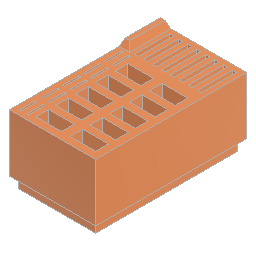
Online-Storage-Carrier (Autodesk Fusion 360 design; units mm, degrees)
Autodesk Fusion 360 part; units mm, degrees
sketch "Sketch1" plane through (0, 0, 18.175) normal (0, 0, 1) x (-1, 0, 0)
  line L0 (-2.95, 294.992) -> (-2.95, 195.892)
  line L1 (-2.95, 195.892) -> (-57.05, 195.892)
  line L2 (-57.05, 195.892) -> (-57.05, 294.992)
  line L3 (-57.05, 294.992) -> (-2.95, 294.992)
  line L4 (0, 192.942) -> (0, 297.942)
  line L5 (0, 297.942) -> (-60, 297.942)
  line L6 (-60, 297.942) -> (-60, 192.942)
  line L7 (-60, 192.942) -> (0, 192.942)
  line L8 (0, 297.942) -> (-60, 297.942)
  line L9 (-60, 297.942) -> (-60, 192.942)
  line L10 (-60, 192.942) -> (0, 192.942)
  line L11 (0, 192.942) -> (0, 297.942)
  line L12 (-56.95, 294.892) -> (-56.95, 195.992)
  line L13 (-56.95, 195.992) -> (-3.05, 195.992)
  line L14 (-3.05, 195.992) -> (-3.05, 294.892)
  line L15 (-3.05, 294.892) -> (-56.95, 294.892)
  point P0 (0, 297.942)
  dimension "d14" = 60
  dimension "d15" = 105
  dimension "d17" = 0.1
  constraint horizontal L8
  constraint vertical L9
  constraint horizontal L10
  constraint vertical L11
  constraint coincident P0 L4.end
  measures "d14" distance of P0 L5.end
  measures "d15" distance of P0 L4.start
  measures "d17" distance of L0 L14
extrude "Extrude1" add sketch "Sketch1" against normal blind 7.5 contours L12 L13 L14 L15
sketch "Sketch2" plane through (0, 0, 18.175) normal (0, 0, 1) x (-1, 0, 0)
  line L0 (-3.05, 294.892) -> (-56.95, 294.892)
  line L1 (-56.95, 294.892) -> (-56.95, 195.992)
  line L2 (-56.95, 195.992) -> (-3.05, 195.992)
  line L3 (-3.05, 195.992) -> (-3.05, 294.892)
  line L4 (0, 297.942) -> (-60, 297.942)
  line L5 (-60, 297.942) -> (-60, 192.942)
  line L6 (-60, 192.942) -> (0, 192.942)
  line L7 (0, 192.942) -> (0, 297.942)
  point P0 (0, 297.942)
  dimension "d21" = 60
  dimension "d22" = 105
  constraint horizontal L4
  constraint vertical L5
  constraint horizontal L6
  constraint vertical L7
  constraint coincident P0 L4.start
  measures "d21" distance of P0 L4.end
  measures "d22" distance of P0 L6.end
extrude "Extrude2" add sketch "Sketch2" along normal blind 40 contours L0 L1 L2 L3 | L4 L5 L6 L7
sketch "Sketch3" plane through (0, 0, 58.175) normal (0, 0, 1) x (-1, 0, 0)
  line L0 (0, 192.942) -> (0, 297.942)
  line L1 (0, 297.942) -> (-60, 297.942)
  line L2 (-60, 297.942) -> (-60, 192.942)
  line L3 (-60, 192.942) -> (0, 192.942)
  line L4 (-55, 284.142) -> (-37.2, 284.142)
  line L5 (-37.2, 284.142) -> (-37.2, 292.942)
  line L6 (-37.2, 292.942) -> (-55, 292.942)
  line L7 (-55, 292.942) -> (-55, 284.142)
  line L8 (-60, 224.192) -> (0, 224.192)
  line L9 (-55, 270.342) -> (-37.2, 270.342)
  line L10 (-37.2, 270.342) -> (-37.2, 279.142)
  line L11 (-37.2, 279.142) -> (-55, 279.142)
  line L12 (-55, 279.142) -> (-55, 270.342)
  line L13 (-55, 256.542) -> (-37.2, 256.542)
  line L14 (-37.2, 256.542) -> (-37.2, 265.342)
  line L15 (-37.2, 265.342) -> (-55, 265.342)
  line L16 (-55, 265.342) -> (-55, 256.542)
  line L17 (-55, 242.742) -> (-37.2, 242.742)
  line L18 (-37.2, 242.742) -> (-37.2, 251.542)
  line L19 (-37.2, 251.542) -> (-55, 251.542)
  line L20 (-55, 251.542) -> (-55, 242.742)
  line L21 (-55, 228.942) -> (-37.2, 228.942)
  line L22 (-37.2, 228.942) -> (-37.2, 237.742)
  line L23 (-37.2, 237.742) -> (-55, 237.742)
  line L24 (-55, 237.742) -> (-55, 228.942)
  line L25 (-31.2, 284.142) -> (-13.4, 284.142)
  line L26 (-13.4, 284.142) -> (-13.4, 292.942)
  line L27 (-13.4, 292.942) -> (-31.2, 292.942)
  line L28 (-31.2, 292.942) -> (-31.2, 284.142)
  line L29 (-31.2, 270.342) -> (-13.4, 270.342)
  line L30 (-13.4, 270.342) -> (-13.4, 279.142)
  line L31 (-13.4, 279.142) -> (-31.2, 279.142)
  line L32 (-31.2, 279.142) -> (-31.2, 270.342)
  line L33 (-31.2, 256.542) -> (-13.4, 256.542)
  line L34 (-13.4, 256.542) -> (-13.4, 265.342)
  line L35 (-13.4, 265.342) -> (-31.2, 265.342)
  line L36 (-31.2, 265.342) -> (-31.2, 256.542)
  line L37 (-31.2, 242.742) -> (-13.4, 242.742)
  line L38 (-13.4, 242.742) -> (-13.4, 251.542)
  line L39 (-13.4, 251.542) -> (-31.2, 251.542)
  line L40 (-31.2, 251.542) -> (-31.2, 242.742)
  line L41 (-31.2, 228.942) -> (-13.4, 228.942)
  line L42 (-13.4, 228.942) -> (-13.4, 237.742)
  line L43 (-13.4, 237.742) -> (-31.2, 237.742)
  line L44 (-31.2, 237.742) -> (-31.2, 228.942)
  dimension "d33" = 17.8
  dimension "d34" = 8.8
  dimension "d35" = 5
  dimension "d36" = 5
  dimension "d38" = 73.75
  dimension "d39" = 31.25
  dimension "d42" = 13.8
  dimension "d43" = 23.8
  dimension "d44" = 4.75
  dimension "d45" = 5
  dimension "d46" = 6
  constraint horizontal L4
  constraint vertical L5
  constraint horizontal L6
  constraint vertical L7
  constraint coincident L2 L8.start
  constraint coincident L0 L8.end
  constraint perpendicular L0 L8
  measures "d33" distance of L4.start L4.end
  measures "d34" distance of L4.start L6.end
  measures "d35" distance of L1 L6
  measures "d36" distance of L2 L7
  measures "d38" distance of L1 L8
  measures "d39" distance of L3 L8
  measures "d44" distance of L8 L21
  measures "d45" distance of L17 L23
  measures "d46" distance of L22 L44
extrude "Extrude3" cut sketch "Sketch3" against normal blind 37.5 contours L4 L5 L6 L7 | L9 L10 L11 L12 | L13 L14 L15 L16 | L17 L18 L19 L20 | L21 L22 L23 L24 | L25 L26 L27 L28 | L29 L30 L31 L32 | L33 L34 L35 L36 | L37 L38 L39 L40 | L41 L42 L43 L44
sketch "Sketch4" plane through (0, 0, 58.175) normal (0, 0, 1) x (-1, 0, 0)
  line L0 (-37.2, 242.742) -> (-55, 242.742)
  line L1 (-55, 242.742) -> (-55, 251.542)
  line L2 (-55, 251.542) -> (-37.2, 251.542)
  line L3 (-37.2, 251.542) -> (-37.2, 242.742)
  line L4 (-37.2, 270.342) -> (-55, 270.342)
  line L5 (-55, 270.342) -> (-55, 279.142)
  line L6 (-55, 279.142) -> (-37.2, 279.142)
  line L7 (-37.2, 279.142) -> (-37.2, 270.342)
  line L8 (-37.2, 284.142) -> (-55, 284.142)
  line L9 (-55, 284.142) -> (-55, 292.942)
  line L10 (-55, 292.942) -> (-37.2, 292.942)
  line L11 (-37.2, 292.942) -> (-37.2, 284.142)
  line L12 (-37.2, 256.542) -> (-55, 256.542)
  line L13 (-55, 256.542) -> (-55, 265.342)
  line L14 (-55, 265.342) -> (-37.2, 265.342)
  line L15 (-37.2, 265.342) -> (-37.2, 256.542)
  line L16 (-37.2, 228.942) -> (-55, 228.942)
  line L17 (-55, 228.942) -> (-55, 237.742)
  line L18 (-55, 237.742) -> (-37.2, 237.742)
  line L19 (-37.2, 237.742) -> (-37.2, 228.942)
  line L20 (-13.4, 242.742) -> (-31.2, 242.742)
  line L21 (-31.2, 242.742) -> (-31.2, 251.542)
  line L22 (-31.2, 251.542) -> (-13.4, 251.542)
  line L23 (-13.4, 251.542) -> (-13.4, 242.742)
  line L24 (-13.4, 270.342) -> (-31.2, 270.342)
  line L25 (-31.2, 270.342) -> (-31.2, 279.142)
  line L26 (-31.2, 279.142) -> (-13.4, 279.142)
  line L27 (-13.4, 279.142) -> (-13.4, 270.342)
  line L28 (-13.4, 284.142) -> (-31.2, 284.142)
  line L29 (-31.2, 284.142) -> (-31.2, 292.942)
  line L30 (-31.2, 292.942) -> (-13.4, 292.942)
  line L31 (-13.4, 292.942) -> (-13.4, 284.142)
  line L32 (-13.4, 256.542) -> (-31.2, 256.542)
  line L33 (-31.2, 256.542) -> (-31.2, 265.342)
  line L34 (-31.2, 265.342) -> (-13.4, 265.342)
  line L35 (-13.4, 265.342) -> (-13.4, 256.542)
  line L36 (-13.4, 228.942) -> (-31.2, 228.942)
  line L37 (-31.2, 228.942) -> (-31.2, 237.742)
  line L38 (-31.2, 237.742) -> (-13.4, 237.742)
  line L39 (-13.4, 237.742) -> (-13.4, 228.942)
  line L40 (0, 192.942) -> (0, 297.942)
  line L41 (0, 297.942) -> (-60, 297.942)
  line L42 (-60, 297.942) -> (-60, 192.942)
  line L43 (-60, 192.942) -> (0, 192.942)
  line L44 (-53.75, 196.442) -> (-56.5, 196.442)
  line L45 (-56.5, 196.442) -> (-56.5, 220.942)
  line L46 (-56.5, 220.942) -> (-53.75, 220.942)
  line L47 (-53.75, 220.942) -> (-53.75, 196.442)
  line L48 (-47.5, 196.442) -> (-50.25, 196.442)
  line L49 (-47.5, 220.942) -> (-47.5, 196.442)
  line L50 (-50.25, 196.442) -> (-50.25, 220.942)
  line L51 (-50.25, 220.942) -> (-47.5, 220.942)
  line L52 (-41.25, 196.442) -> (-44, 196.442)
  line L53 (-41.25, 220.942) -> (-41.25, 196.442)
  line L54 (-44, 196.442) -> (-44, 220.942)
  line L55 (-44, 220.942) -> (-41.25, 220.942)
  line L56 (-35, 196.442) -> (-37.75, 196.442)
  line L57 (-35, 220.942) -> (-35, 196.442)
  line L58 (-37.75, 196.442) -> (-37.75, 220.942)
  line L59 (-37.75, 220.942) -> (-35, 220.942)
  line L60 (-28.75, 196.442) -> (-31.5, 196.442)
  line L61 (-28.75, 220.942) -> (-28.75, 196.442)
  line L62 (-31.5, 196.442) -> (-31.5, 220.942)
  line L63 (-31.5, 220.942) -> (-28.75, 220.942)
  line L64 (-22.5, 196.442) -> (-25.25, 196.442)
  line L65 (-22.5, 220.942) -> (-22.5, 196.442)
  line L66 (-25.25, 196.442) -> (-25.25, 220.942)
  line L67 (-25.25, 220.942) -> (-22.5, 220.942)
  line L68 (-16.25, 196.442) -> (-19, 196.442)
  line L69 (-16.25, 220.942) -> (-16.25, 196.442)
  line L70 (-19, 196.442) -> (-19, 220.942)
  line L71 (-19, 220.942) -> (-16.25, 220.942)
  line L72 (-10, 196.442) -> (-12.75, 196.442)
  line L73 (-10, 220.942) -> (-10, 196.442)
  line L74 (-12.75, 196.442) -> (-12.75, 220.942)
  line L75 (-12.75, 220.942) -> (-10, 220.942)
  dimension "d51" = 2.75
  dimension "d52" = 24.5
  dimension "d54" = 3.5
  dimension "d55" = 3.5
  dimension "d65" = 6.25
  dimension "d66" = 0
  constraint horizontal L44
  constraint vertical L45
  constraint horizontal L46
  constraint vertical L47
  measures "d51" distance of L44.start L44.end
  measures "d52" distance of L44.start L46.end
  measures "d54" distance of L43 L44
  measures "d55" distance of L42 L45
sketch "Sketch5" plane through (0, 0, 58.175) normal (0, 0, 1) x (-1, 0, 0)
  line L0 (-37.2, 242.742) -> (-55, 242.742)
  line L1 (-55, 242.742) -> (-55, 251.542)
  line L2 (-55, 251.542) -> (-37.2, 251.542)
  line L3 (-37.2, 251.542) -> (-37.2, 242.742)
  line L4 (-37.2, 270.342) -> (-55, 270.342)
  line L5 (-55, 270.342) -> (-55, 279.142)
  line L6 (-55, 279.142) -> (-37.2, 279.142)
  line L7 (-37.2, 279.142) -> (-37.2, 270.342)
  line L8 (-37.2, 284.142) -> (-55, 284.142)
  line L9 (-55, 284.142) -> (-55, 292.942)
  line L10 (-55, 292.942) -> (-37.2, 292.942)
  line L11 (-37.2, 292.942) -> (-37.2, 284.142)
  line L12 (-37.2, 256.542) -> (-55, 256.542)
  line L13 (-55, 256.542) -> (-55, 265.342)
  line L14 (-55, 265.342) -> (-37.2, 265.342)
  line L15 (-37.2, 265.342) -> (-37.2, 256.542)
  line L16 (-37.2, 228.942) -> (-55, 228.942)
  line L17 (-55, 228.942) -> (-55, 237.742)
  line L18 (-55, 237.742) -> (-37.2, 237.742)
  line L19 (-37.2, 237.742) -> (-37.2, 228.942)
  line L20 (-13.4, 242.742) -> (-31.2, 242.742)
  line L21 (-31.2, 242.742) -> (-31.2, 251.542)
  line L22 (-31.2, 251.542) -> (-13.4, 251.542)
  line L23 (-13.4, 251.542) -> (-13.4, 242.742)
  line L24 (-13.4, 270.342) -> (-31.2, 270.342)
  line L25 (-31.2, 270.342) -> (-31.2, 279.142)
  line L26 (-31.2, 279.142) -> (-13.4, 279.142)
  line L27 (-13.4, 279.142) -> (-13.4, 270.342)
  line L28 (-13.4, 284.142) -> (-31.2, 284.142)
  line L29 (-31.2, 284.142) -> (-31.2, 292.942)
  line L30 (-31.2, 292.942) -> (-13.4, 292.942)
  line L31 (-13.4, 292.942) -> (-13.4, 284.142)
  line L32 (-13.4, 256.542) -> (-31.2, 256.542)
  line L33 (-31.2, 256.542) -> (-31.2, 265.342)
  line L34 (-31.2, 265.342) -> (-13.4, 265.342)
  line L35 (-13.4, 265.342) -> (-13.4, 256.542)
  line L36 (-13.4, 228.942) -> (-31.2, 228.942)
  line L37 (-31.2, 228.942) -> (-31.2, 237.742)
  line L38 (-31.2, 237.742) -> (-13.4, 237.742)
  line L39 (-13.4, 237.742) -> (-13.4, 228.942)
  line L40 (0, 192.942) -> (0, 297.942)
  line L41 (0, 297.942) -> (-60, 297.942)
  line L42 (-60, 297.942) -> (-60, 192.942)
  line L43 (-60, 192.942) -> (0, 192.942)
  line L44 (0, 192.942) -> (-7.25, 192.942)
  line L45 (-7.25, 192.942) -> (-7.25, 221.442)
  line L46 (-7.25, 221.442) -> (0, 221.442)
  line L47 (0, 221.442) -> (0, 192.942)
  dimension "d56" = 7.25
  dimension "d57" = 28.5
  constraint horizontal L44
  constraint vertical L45
  constraint horizontal L46
  constraint vertical L47
  constraint coincident L40.start L43.end
  measures "d56" distance of L40.start L44.end
  measures "d57" distance of L40.start L46.end
extrude "Extrude4" add sketch "Sketch5" along normal blind 3 contours L40 L43 L44 L45 L46 L47
chamfer "Chamfer1" distance 4 distance2 3 2 edges at (7.25, -207.192, 61.175) (3.625, -221.442, 61.175) measured on face at (2.4167, -211.942, 61.175) measured on face at (2.4167, -211.942, 61.175)
extrude "Extrude5" cut sketch "Sketch4" against normal blind 21 contours L44 L45 L46 L47 | L48 L49 L50 L51 | L52 L53 L54 L55 | L56 L57 L58 L59 | L60 L61 L62 L63 | L64 L65 L66 L67 | L68 L69 L70 L71 | L72 L73 L74 L75
sketch "Sketch1 (2)" plane through (0, 0, 58.175) normal (0, 0, 1) x (-1, 0, 0)
  line L0 (-22.5, 196.442) -> (-25.25, 196.442)
  line L1 (-25.25, 196.442) -> (-25.25, 220.942)
  line L2 (-25.25, 220.942) -> (-22.5, 220.942)
  line L3 (-22.5, 220.942) -> (-22.5, 196.442)
  line L4 (-47.5, 196.442) -> (-50.25, 196.442)
  line L5 (-50.25, 196.442) -> (-50.25, 220.942)
  line L6 (-50.25, 220.942) -> (-47.5, 220.942)
  line L7 (-47.5, 220.942) -> (-47.5, 196.442)
  line L8 (-41.25, 196.442) -> (-44, 196.442)
  line L9 (-44, 196.442) -> (-44, 220.942)
  line L10 (-44, 220.942) -> (-41.25, 220.942)
  line L11 (-41.25, 220.942) -> (-41.25, 196.442)
  line L12 (-16.25, 196.442) -> (-19, 196.442)
  line L13 (-19, 196.442) -> (-19, 220.942)
  line L14 (-19, 220.942) -> (-16.25, 220.942)
  line L15 (-16.25, 220.942) -> (-16.25, 196.442)
  line L16 (-28.75, 196.442) -> (-31.5, 196.442)
  line L17 (-31.5, 196.442) -> (-31.5, 220.942)
  line L18 (-31.5, 220.942) -> (-28.75, 220.942)
  line L19 (-28.75, 220.942) -> (-28.75, 196.442)
  line L20 (-56.5, 196.442) -> (-56.5, 220.942)
  line L21 (-56.5, 220.942) -> (-53.75, 220.942)
  line L22 (-53.75, 220.942) -> (-53.75, 196.442)
  line L23 (-53.75, 196.442) -> (-56.5, 196.442)
  line L24 (-35, 196.442) -> (-37.75, 196.442)
  line L25 (-37.75, 196.442) -> (-37.75, 220.942)
  line L26 (-37.75, 220.942) -> (-35, 220.942)
  line L27 (-35, 220.942) -> (-35, 196.442)
  line L28 (-10, 196.442) -> (-12.75, 196.442)
  line L29 (-12.75, 196.442) -> (-12.75, 220.942)
  line L30 (-12.75, 220.942) -> (-10, 220.942)
  line L31 (-10, 220.942) -> (-10, 196.442)
  line L32 (-7.25, 192.942) -> (-7.25, 221.442)
  line L33 (-7.25, 221.442) -> (0, 221.442)
  line L34 (0, 221.442) -> (0, 297.942)
  line L35 (0, 297.942) -> (-60, 297.942)
  line L36 (-60, 297.942) -> (-60, 192.942)
  line L37 (-60, 192.942) -> (-7.25, 192.942)
  line L38 (-13.4, 228.942) -> (-31.2, 228.942)
  line L39 (-31.2, 228.942) -> (-31.2, 237.742)
  line L40 (-31.2, 237.742) -> (-13.4, 237.742)
  line L41 (-13.4, 237.742) -> (-13.4, 228.942)
  line L42 (-13.4, 256.542) -> (-31.2, 256.542)
  line L43 (-31.2, 256.542) -> (-31.2, 265.342)
  line L44 (-31.2, 265.342) -> (-13.4, 265.342)
  line L45 (-13.4, 265.342) -> (-13.4, 256.542)
  line L46 (-13.4, 284.142) -> (-31.2, 284.142)
  line L47 (-31.2, 284.142) -> (-31.2, 292.942)
  line L48 (-31.2, 292.942) -> (-13.4, 292.942)
  line L49 (-13.4, 292.942) -> (-13.4, 284.142)
  line L50 (-13.4, 270.342) -> (-31.2, 270.342)
  line L51 (-31.2, 270.342) -> (-31.2, 279.142)
  line L52 (-31.2, 279.142) -> (-13.4, 279.142)
  line L53 (-13.4, 279.142) -> (-13.4, 270.342)
  line L54 (-13.4, 242.742) -> (-31.2, 242.742)
  line L55 (-31.2, 242.742) -> (-31.2, 251.542)
  line L56 (-31.2, 251.542) -> (-13.4, 251.542)
  line L57 (-13.4, 251.542) -> (-13.4, 242.742)
  line L58 (-37.2, 228.942) -> (-55, 228.942)
  line L59 (-55, 228.942) -> (-55, 237.742)
  line L60 (-55, 237.742) -> (-37.2, 237.742)
  line L61 (-37.2, 237.742) -> (-37.2, 228.942)
  line L62 (-37.2, 256.542) -> (-55, 256.542)
  line L63 (-55, 256.542) -> (-55, 265.342)
  line L64 (-55, 265.342) -> (-37.2, 265.342)
  line L65 (-37.2, 265.342) -> (-37.2, 256.542)
  line L66 (-37.2, 284.142) -> (-55, 284.142)
  line L67 (-55, 284.142) -> (-55, 292.942)
  line L68 (-55, 292.942) -> (-37.2, 292.942)
  line L69 (-37.2, 292.942) -> (-37.2, 284.142)
  line L70 (-37.2, 270.342) -> (-55, 270.342)
  line L71 (-55, 270.342) -> (-55, 279.142)
  line L72 (-55, 279.142) -> (-37.2, 279.142)
  line L73 (-37.2, 279.142) -> (-37.2, 270.342)
  line L74 (-37.2, 242.742) -> (-55, 242.742)
  line L75 (-55, 242.742) -> (-55, 251.542)
  line L76 (-55, 251.542) -> (-37.2, 251.542)
  line L77 (-37.2, 251.542) -> (-37.2, 242.742)
  line L78 (-9.8, 294.342) -> (-8.5, 294.342)
  line L79 (-8.5, 294.342) -> (-8.5, 283.092)
  line L80 (-8.5, 283.092) -> (-9.8, 283.092)
  line L81 (-9.8, 283.092) -> (-9.8, 294.342)
  line L82 (-3.6, 294.342) -> (-3.6, 283.092)
  line L83 (-3.6, 283.092) -> (-4.9, 283.092)
  line L84 (-4.9, 283.092) -> (-4.9, 294.342)
  line L85 (-4.9, 294.342) -> (-3.6, 294.342)
  line L86 (-8.5, 279.492) -> (-8.5, 268.242)
  line L87 (-8.5, 268.242) -> (-9.8, 268.242)
  line L88 (-9.8, 268.242) -> (-9.8, 279.492)
  line L89 (-9.8, 279.492) -> (-8.5, 279.492)
  line L90 (-3.6, 279.492) -> (-3.6, 268.242)
  line L91 (-3.6, 268.242) -> (-4.9, 268.242)
  line L92 (-4.9, 268.242) -> (-4.9, 279.492)
  line L93 (-4.9, 279.492) -> (-3.6, 279.492)
  line L94 (-8.5, 264.642) -> (-8.5, 253.392)
  line L95 (-8.5, 253.392) -> (-9.8, 253.392)
  line L96 (-9.8, 253.392) -> (-9.8, 264.642)
  line L97 (-9.8, 264.642) -> (-8.5, 264.642)
  line L98 (-3.6, 264.642) -> (-3.6, 253.392)
  line L99 (-3.6, 253.392) -> (-4.9, 253.392)
  line L100 (-4.9, 253.392) -> (-4.9, 264.642)
  line L101 (-4.9, 264.642) -> (-3.6, 264.642)
  line L102 (-8.5, 249.792) -> (-8.5, 238.542)
  line L103 (-8.5, 238.542) -> (-9.8, 238.542)
  line L104 (-9.8, 238.542) -> (-9.8, 249.792)
  line L105 (-9.8, 249.792) -> (-8.5, 249.792)
  line L106 (-3.6, 249.792) -> (-3.6, 238.542)
  line L107 (-3.6, 238.542) -> (-4.9, 238.542)
  line L108 (-4.9, 238.542) -> (-4.9, 249.792)
  line L109 (-4.9, 249.792) -> (-3.6, 249.792)
  line L110 (-8.5, 234.942) -> (-8.5, 223.692)
  line L111 (-8.5, 223.692) -> (-9.8, 223.692)
  line L112 (-9.8, 223.692) -> (-9.8, 234.942)
  line L113 (-9.8, 234.942) -> (-8.5, 234.942)
  line L114 (-3.6, 234.942) -> (-3.6, 223.692)
  line L115 (-3.6, 223.692) -> (-4.9, 223.692)
  line L116 (-4.9, 223.692) -> (-4.9, 234.942)
  line L117 (-4.9, 234.942) -> (-3.6, 234.942)
  dimension "d71" = 1.3
  dimension "d72" = 11.25
  dimension "d73" = 13.4
  dimension "d75" = 3.6
  dimension "d76" = 3.6
  dimension "d80" = 4.9
  dimension "d81" = -14.85
  constraint horizontal L78
  constraint vertical L79
  constraint horizontal L80
  constraint vertical L81
  measures "d71" distance of L78.start L78.end
  measures "d72" distance of L78.start L80.end
  measures "d73" distance of L34 L49
  measures "d75" distance of L49 L81
  measures "d76" distance of L35 L78
extrude "Extrude6" cut sketch "Sketch1 (2)" against normal blind 9.5 contours L78 L79 L80 L81 | L82 L83 L84 L85 | L86 L87 L88 L89 | L90 L91 L92 L93 | L94 L95 L96 L97 | L98 L99 L100 L101 | L102 L103 L104 L105 | L106 L107 L108 L109 | L110 L111 L112 L113 | L114 L115 L116 L117
equation "d14 = OnlineStorageWidth"
equation "d15 = OnlineStorageLength"
equation "d16 = -HoldersterWallWidth - SmallTolerence"
equation "d19 = -InsertLockDepth"
equation "d21 = OnlineStorageWidth"
equation "d22 = OnlineStorageLength"
equation "d24 = OnlineStorageHeight"
equation "d33 = OnlineStorageUSBWidth"
equation "d34 = OnlineStorageUSBLength"
equation "d35 = OnlineStorageUSBSpace"
equation "d36 = OnlineStorageUSBSpace"
equation "d38 = OnlineStorageLength - OnlineStorageUSBAreaLength"
equation "d42 = OnlineStorageUSBLength + OnlineStorageUSBSpace"
equation "d43 = OnlineStorageUSBWidth + ( OnlineStorageUSBSpace * 1.2 )"
equation "d49 = -OnlineStorageUSBDepth"
equation "d51 = OnlineStorageSDWidth"
equation "d52 = OnlineStorageSDLength"
equation "d54 = OnlineStorageSDSpace"
equation "d55 = OnlineStorageSDSpace"
equation "d63 = OnlineStorageSDAmount"
equation "d65 = OnlineStorageSDWidth + OnlineStorageSDSpace"
equation "d69 = -OnlineStorageSDDepth"
equation "d71 = OnlineStorageMSDWidth"
equation "d72 = OnlineStorageMSDLength"
equation "d75 = OnlineStorageMSDSpace"
equation "d76 = OnlineStorageMSDSpace"
equation "d80 = OnlineStorageMSDWidth + OnlineStorageMSDSpace"
equation "d81 = -OnlineStorageMSDLength - ( OnlineStorageMSDSpace * 1 )"
equation "d84 = -OnlineStorageMSDDepth"
equation "SmallTolerence = 0.05 mm"
equation "HoldersterWallWidth = 3 mm"
equation "OnlineStorageLength = 105 mm"
equation "OnlineStorageWidth = 60 mm"
equation "InsertLockDepth = 7.5 mm"
equation "OnlineStorageHeight = 40 mm"
equation "OnlineStorageUSBWidth = 17.8 mm"
equation "OnlineStorageUSBLength = 8.8 mm"
equation "OnlineStorageSDLength = 24.5 mm"
equation "OnlineStorageSDWidth = 2.75 mm"
equation "OnlineStorageMSDLength = 11.25 mm"
equation "OnlineStorageMSDWidth = 1.25 mm + SmallTolerence"
equation "OnlineStorageUSBSpace = 5 mm"
equation "OnlineStorageUSBAreaLength = 31.25 mm"
equation "OnlineStorageUSBDepth = 37.5 mm"
equation "OnlineStorageSDSpace = 3.5 mm"
equation "OnlineStorageSDAreaLength = OnlineStorageWidth - d56"
equation "OnlineStorageSDAmount = floor(( OnlineStorageSDAreaLength ) / ( OnlineStorageSDWidth + OnlineStorageSDSpace ))"
equation "OnlineStorageSDDepth = 21 mm"
equation "OnlineStorageMSDSpace = 3.6 mm"
equation "OnlineStorageMSDDepth = 9.5 mm"
